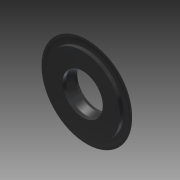
# Autodesk Inventor part: A1169970081
Saved by Autodesk Inventor 2014 SP2 (Build 180246200, 246)
## iProperties
Created: 2015-12-21
Part Number: A1169970081
Material: Rubber, Silicone
Document SubType Name: Modeling
Designer: Lukasz Szmit
Density: 1.25 g/cm^3
Appearance: Rubber - Black - Version 1.1
Author: Lukasz Szmit
Autodesk Inventor part; units mm, degrees
ref_plane "YZ Plane" through (0, 0, 0) normal (1, 0, 0) x (0, 1, 0)
ref_plane "XZ Plane" through (0, 0, 0) normal (0, 1, 0) x (-1, 0, 0)
ref_plane "XY Plane" through (0, 0, 0) normal (0, 0, 1) x (1, 0, 0)
sketch "Sketch6" plane through (0, 0, 0) normal (0, 0, 1) x (1, 0, 0)
  line L0 (0, 15) -> (0, 0)
  line L1 (-32, 0) -> (-32, -3)
  line L2 (-32, -3) -> (-17.25, -3)
  line L3 (-17.25, 0) -> (-19.9798, 0)
  line L4 (-32, 0) -> (-29, 0)
  line L5 (-29, 0) -> (-29, 1)
  line L6 (-19.9798, 0) -> (-17.25, 7.5001)
  line L7 (-20.037, 7.3286) -> (-30.8443, 4.9723)
  line L8 (-17.25, 7.5001) -> (-17.25, 9.5001)
  line L9 (-17.25, 9.5001) -> (-19.25, 9.5001)
  line L10 (-19.25, 9.5001) -> (-19.25, 8.3056)
  arc A0 (-20.037, 7.3286) -> (-19.25, 8.3056) centre (-20.25, 8.3056) ccw
  line L11 (-17.25, 0) -> (-17.25, -3)
  line L12 (-38.7845, 0.5) -> (-36.7845, 0.5)
  line L13 (-29, 1) -> (-32, 1)
  arc A1 (-32, 1) -> (-36.7845, 0.5) centre (-32.4339, -17.9895) ccw
  arc A2 (-30.8443, 4.9723) -> (-38.7845, 0.5) centre (-28.7158, -8.0913) ccw
  point P0 (0, 0)
  point P1 (-19.25, 7.5001)
  dimension "d30" = 17.25
  dimension "d56" = 2
  dimension "d74" = 17.25
  dimension "d75" = 1
  dimension "d76" = 2
  dimension "d77" = 3
  dimension "d78" = 3
  dimension "d79" = 1
  dimension "d80" = 29
  dimension "d81" = 2
  dimension "d82" = 3
  dimension "d84" = 70
  dimension "d85" = 0.5
  constraints: 28 end point, 7 perpendicular, 6 point on circle, 3 centre point, 2 point on line, 2 tangent, 1 vertical
  measures "d30" distance of L3.start point (0, 0)
  measures "d56" distance of L6.end point (-19.25, 7.5)
  measures "d74" horizontal distance of point (0, 0) L6.end
  measures "d75" radius of A0
  measures "d76" distance of L6.end L8.end
  measures "d77" distance of L1.start L1.end
  measures "d78" distance of L1.start L4.end
  measures "d79" distance of L4.end L5.end
  measures "d80" distance of L0.end L4.end
  measures "d81" distance of L12.start L12.end
  measures "d82" distance of L5.end L13.end
  measures "d84" angle of L6 L3
  measures "d85" distance between parallel lines of L12 L4
revolve "Revolution2" add sketch "Sketch6" angle 360 about axis through (0, 15, 0) along (0, -1, 0)
equation "\"d56\" = d76"
equation "\"d74\" = d30"
equation "\"d77\" = d78"
equation "\"d81\" = d56"
equation "\"d82\" = d78"
equation "\"d85\" = 0.5 * d79"
body "Solid2"
